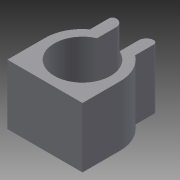
# Autodesk Inventor part: WireClip
Saved by Autodesk Inventor 2015 SP1 (Build 190203100, 203)
## iProperties
Created: 2015-04-12
Part Number: WireClip
Material: Generic
Document SubType Name: Modeling
Designer: Jack
Density: 1 g/cm^3
Appearance: Default
Author: Jack
Autodesk Inventor part; units mm, degrees
ref_plane "YZ Plane" through (0, 0, 0) normal (1, 0, 0) x (0, 1, 0)
ref_plane "XZ Plane" through (0, 0, 0) normal (0, 1, 0) x (-1, 0, 0)
ref_plane "XY Plane" through (0, 0, 0) normal (0, 0, 1) x (1, 0, 0)
sketch "Sketch3" plane through (0, 0, 0) normal (0, 0, 1) x (1, 0, 0)
  line L0 (0, 0) -> (-5, 0)
  line L1 (-5, 0) -> (-5, 5)
  line L2 (0, 0) -> (5, 0)
  line L3 (5, 0) -> (5, 5)
  arc A0 (-1.5, 8.4369) -> (1.5, 8.4369) centre (0, 5) ccw
  line L4 (-3, 9) -> (-3, 12)
  line L5 (-3, 12) -> (-1.5, 12)
  line L6 (-1.5, 12) -> (-1.5, 9.7697)
  line L7 (1.5, 9.7697) -> (1.5, 12)
  line L8 (1.5, 12) -> (3, 12)
  line L9 (3, 12) -> (3, 9)
  line L10 (-1.5, 9.7697) -> (-1.5, 8.4369)
  line L11 (1.5, 9.7697) -> (1.5, 8.4369)
  arc A1 (-3, 9) -> (-5, 5) centre (0, 5) ccw
  arc A2 (5, 5) -> (3, 9) centre (0, 5) ccw
  dimension "d9" = 5
  dimension "d10" = 7.5
  dimension "d11" = 3
  dimension "d12" = 7
  dimension "d13" = 1.5
  dimension "d14" = 5
  dimension "d15" = 5
  dimension "d16" = 1.5
  constraints: 24 end point, 6 point on circle, 4 perpendicular, 4 tangent, 3 centre point, 3 point on line, 2 equal length, 2 parallel, 2 vertical, 1 coincident, 1 horizontal, 1 vertical alignment
  measures "d9" distance of L0.start A1.centre
  measures "d10" diameter of A0
  measures "d11" distance between parallel lines of L7 L6
  measures "d12" distance from line of A1.centre L8
  measures "d13" distance of L7.end L8.end
  measures "d14" radius of A1
  measures "d15" radius of A2
  measures "d16" distance from line of A1.centre L7
extrude "Extrusion1" add sketch "Sketch3" along normal blind 8
fillet "Fillet1" radius 1 2 edges at (-1.5, 12, 4) (1.5, 12, 4)
fillet "Fillet2" radius 0.5 2 edges at (3, 12, 4) (-3, 12, 4)
body "Solid1"
